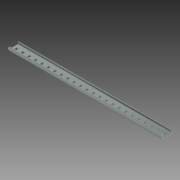
# Autodesk Inventor part: 276-1926
Saved by Autodesk Inventor 2016 SP2 (Build 200236200, 236)
## iProperties
Category: Motion
Company: Autodesk Inc.
Created: 2012-02-22
Part Number: 276-1926
Material: Steel
Document SubType Name: Sheet Metal
Designer: Autodesk Inc.
Density: 7.85 g/cm^3
Sheet Metal Rule: Default
Catalog Web Link: http://www.vexrobotics.com/276-1926.html
Vendor: VEX
Mass: 122.945 g
Surface Area: 281.051 cm^2
Volume: 15.6618 cm^3
Appearance: Zinc
Author: Autodesk Inc.
Autodesk Inventor part; units mm, degrees
ref_plane "YZ Plane" through (0, 0, 0) normal (1, 0, 0) x (0, 1, 0)
ref_plane "XZ Plane" through (0, 0, 0) normal (0, 1, 0) x (-1, 0, 0)
ref_plane "XY Plane" through (0, 0, 0) normal (0, 0, 1) x (1, 0, 0)
sketch "Sketch1" plane through (0, 0, 0) normal (0, 0, 1) x (1, 0, 0)
  line L0 (0, 0) -> (22.0218, 0)
  line L1 (22.0218, 0) -> (22.0218, 304.8)
  line L2 (22.0218, 304.8) -> (0, 304.8)
  line L3 (0, 304.8) -> (0, 0)
  dimension "d0" = 22.0218
  dimension "d1" = 304.8
  measures "d0" distance of L2.end L1.end
  measures "d1" distance of L1.end L0.end
extrude "Plate1" add sketch "Sketch1" against normal blind 1.1938
sketch "Sketch2" plane through (1.1531, 0, -1.5028) normal (-0.9659258, 0, 0.258819) x (0, -1, 0)
  line L0 (-304.8, 0) -> (0, 0)
  line L1 (0, 0) -> (0, 7.1946)
  line L2 (0, 7.1946) -> (-304.8, 7.1946)
  line L3 (-304.8, 7.1946) -> (-304.8, 0)
  constraints: 6 end point, 1 horizontal, 1 perpendicular, 1 vertical
edge flange "Flange1" height 5.6388 angle 105 thickness 1.1938 bend radius 0.762 thickness toward (-0.9659258, 0, 0.258819) relief straight relief width 1.1938 relief depth 0.5969 corner gap 0.762 corner form 0 edges at (0, 152.4, 0) (22.0218, 152.4, 0) wall of the first edge with corners at (1.1531, 304.8, -1.5028) (1.1531, 0, -1.5028) (3.0152, 0, 5.4467) (3.0152, 304.8, 5.4467)
bend "Bend1"
corner "Corner1"
chamfer "Corner Chamfer1" distance 1.905 angle 45 4 edges at (2.4387, 0, 5.6012) (19.5831, 0, 5.6012) (2.4387, 304.8, 5.6012) (19.5831, 304.8, 5.6012)
sketch "Sketch4" plane through (0, 0, 0) normal (0, 0, 1) x (1, 0, 0)
  line L0 (2.5488, 0) -> (19.473, 0) projected
  line L1 (12.8143, 4.0386) -> (9.2075, 4.0386)
  line L2 (8.6995, 4.5466) -> (8.6995, 8.1534)
  line L3 (9.2075, 8.6614) -> (12.8143, 8.6614)
  line L4 (13.3223, 8.1534) -> (13.3223, 4.5466)
  arc A0 (8.6995, 4.5466) -> (9.2075, 4.0386) centre (9.2075, 4.5466) ccw
  arc A1 (9.2075, 8.6614) -> (8.6995, 8.1534) centre (9.2075, 8.1534) ccw
  arc A2 (13.3223, 8.1534) -> (12.8143, 8.6614) centre (12.8143, 8.1534) ccw
  arc A3 (12.8143, 4.0386) -> (13.3223, 4.5466) centre (12.8143, 4.5466) ccw
  point P0 (0, 0)
  point P1 (13.3223, 4.0386)
  point P2 (8.6995, 8.6614)
  point P3 (8.6995, 4.0386)
  point P4 (13.3223, 8.6614)
  point P5 (11.0109, 4.0386)
  point P6 (11.0109, 0)
  dimension "d16" = 4.6228
  dimension "d19" = 0.508
  dimension "d23" = 4.5466
  constraints: 8 end point, 8 point on circle, 8 point on line, 8 tangent, 4 centre point, 3 equal radius, 2 midpoint, 2 parallel, 2 perpendicular, 1 horizontal, 1 vertical alignment
  measures "d16" distance of point (8.699, 4.039) point (8.699, 8.661)
  measures "d19" radius of A0
  measures "d23" distance from line of A0.centre L0
extrude "Cut1" cut sketch "Sketch4" against normal blind 1.1938
pattern_linear "Rectangular Pattern1" count 35 spacing 12.7 along (0, 1, 0) of "Cut1"
sketch "Sketch5" plane through (0, 0, 0) normal (0, 0, 1) x (1, 0, 0)
  line L0 (8.6995, 4.5466) -> (8.6995, 8.1534) projected
  circle A0 centre (11.0109, 6.35) radius 2.3114
  point P0 (0, 0)
  constraints: 1 centre point, 1 tangent
surface extrude "ExtrusionSrf1" sketch "Sketch5" against normal up to surface (1.1938 mm away) shown no curves A0
pattern_linear "Rectangular Pattern2" count 24 spacing 12.7 along (0, 1, 0) of "ExtrusionSrf1"
equation "\"d17\" = Thickness"
equation "\"d3\" = BendReliefWidth"
equation "\"d4\" = BendReliefDepth"
equation "\"d5\" = MinimumRemnant"
equation "\"d6\" = BendRadius"
equation "\"d9\" = BendRadius"
equation "\"d10\" = CornerReliefSize"
equation "\"d11\" = GapSize"
equation "\"d12\" = JacobiRadiusSize"
equation "\"BendReliefWidth\" = Thickness"
equation "\"BendReliefDepth\" = 0.5 * Thickness"
equation "\"CornerReliefSize\" = 4 * Thickness"
equation "\"MinimumRemnant\" = 2 * Thickness"
equation "\"TransitionRadius\" = BendRadius"
equation "\"JacobiRadiusSize\" = BendRadius"
equation "\"GapSize\" = Thickness"
equation "\"d2\" = BendRadius"
equation "\"Thickness\" = 1.1938"
equation "\"BendRadius\" = 0.762"
body "Solid1"
body "Srf1"
body "Srf2"
body "Srf3"
body "Srf4"
body "Srf5"
body "Srf6"
body "Srf7"
body "Srf8"
body "Srf9"
body "Srf10"
body "Srf11"
body "Srf12"
body "Srf13"
body "Srf14"
body "Srf15"
body "Srf16"
body "Srf17"
body "Srf18"
body "Srf19"
body "Srf20"
body "Srf21"
body "Srf22"
body "Srf23"
body "Srf24"
